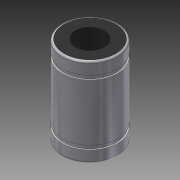
# Autodesk Inventor part: LM08UU
Saved by Autodesk Inventor 2013 (Build 170138000, 138)
## iProperties
Created: 2013-12-30
Part Number: LM08UU
Material: Generic
Document SubType Name: Modeling
Designer: Masta
Density: 1 g/cm^3
Author: Masta
Autodesk Inventor part; units mm, degrees
ref_plane "YZ Plane" through (0, 0, 0) normal (1, 0, 0) x (0, 1, 0)
ref_plane "XZ Plane" through (0, 0, 0) normal (0, 1, 0) x (-1, 0, 0)
ref_plane "XY Plane" through (0, 0, 0) normal (0, 0, 1) x (1, 0, 0)
sketch "Sketch1" plane through (0, 0, 0) normal (0, 0, 1) x (1, 0, 0)
  circle A0 centre (0, 0) radius 4
  circle A1 centre (0, 0) radius 7.5
  circle A2 centre (0, 0) radius 7.15
  dimension "d0" = 8
  dimension "d1" = 15
  dimension "d2" = 14.3
  constraints: 3 centre point, 3 coincident
  measures "d0" diameter of A0
  measures "d1" diameter of A1
  measures "d2" diameter of A2
extrude "Extrusion1" add sketch "Sketch1" along normal blind 4.35 and the other way blind 7.65 contours A1 | A2
extrude "Extrusion2" cut sketch "Sketch1" along normal blind 1.1 contours A1
fillet "Fillet1" radius 0.5 1 edges at (-7.5, 0, 4.35)
mirror "Mirror1" about plane through (0, 0, -7.65) normal (0, 0, -1) of "Extrusion1", "Extrusion2", "Fillet1"
body "Solid1"
